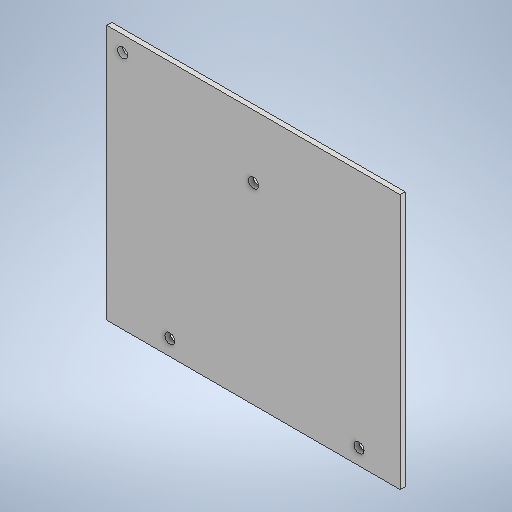
# Autodesk Inventor part: board
Saved by Autodesk Inventor 2026.1 (Build 301233020, 233B)
## iProperties
Created: 2026-02-05
Part Number: board
Material: 一般
Document SubType Name: Modeling
Designer: hibik
Density: 1 g/cm^3
Appearance: 既定
Author: hibik
Autodesk Inventor part; units mm, degrees
ref_plane "YZ Plane" through (0, 0, 0) normal (1, 0, 0) x (0, 1, 0)
ref_plane "XZ Plane" through (0, 0, 0) normal (0, 1, 0) x (-1, 0, 0)
ref_plane "XY Plane" through (0, 0, 0) normal (0, 0, 1) x (1, 0, 0)
sketch "スケッチ1" plane through (0, 0, 0) normal (0, 0, 1) x (1, 0, 0)
  line L0 (46.5, -40.5) -> (-46.5, -40.5)
  line L1 (-46.5, -40.5) -> (-46.5, 40.5)
  line L2 (-46.5, 40.5) -> (46.5, 40.5)
  line L3 (46.5, 40.5) -> (46.5, -40.5)
  line L4 (46.5, -40.5) -> (-46.5, 40.5) construction
  line L5 (-46.5, -40.5) -> (46.5, 40.5) construction
  point P0 (0, 0)
  dimension "d0" = 93
  dimension "d1" = 81
  constraints: 12 end point, 2 midpoint, 2 parallel, 1 horizontal, 1 perpendicular
  measures "d0" distance of L1.end L2.end
  measures "d1" distance of L0.end L1.end
extrude "押し出し1" add sketch "スケッチ1" along normal blind 1.6
sketch "スケッチ2" plane through (0, 0, 1.6) normal (0, 0, 1) x (1, 0, 0)
  circle A0 centre (-41.5, 35.5) radius 1.6
  line L0 (46.5, 40.5) -> (-46.5, 40.5) projected
  line L1 (-46.5, 40.5) -> (-46.5, -40.5) projected
  circle A1 centre (-26.5, -35.5) radius 1.6
  line L2 (-46.5, -40.5) -> (46.5, -40.5) projected
  circle A2 centre (33.5, -35.5) radius 1.6
  circle A3 centre (0, 20.5) radius 1.6
  point P0 (0, 0)
  dimension "d4" = 3.2
  dimension "d5" = 5
  dimension "d6" = 5
  dimension "d7" = 3.2
  dimension "d8" = 20
  dimension "d9" = 5
  dimension "d11" = 80
  dimension "d14" = 20
  constraints: 4 centre point, 2 equal radius, 1 horizontal alignment, 1 vertical alignment
  measures "d4" diameter of A0
  measures "d5" distance from line of L0 A0.centre
  measures "d6" distance from line of L1 A0.centre
  measures "d7" diameter of A1
  measures "d8" distance from line of A1.centre L1
  measures "d9" distance from line of L2 A1.centre
  measures "d11" distance from line of A2.centre L1
  measures "d14" distance from line of L0 A3.centre
extrude "押し出し2" cut sketch "スケッチ2" against normal through all
equation "\"d9\" = d5"
